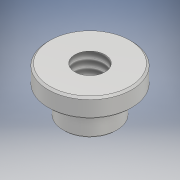
# Autodesk Inventor part: Nut_SMD_M2x0.4_1mm
Saved by Autodesk Inventor 2018 (Build 220112000, 112)
## iProperties
Created: 2018-10-26
Part Number: Nut_SMD_M2x0.4_1mm
Material: Steel, Mild
Description: 9774010243R
Document SubType Name: Modeling
Designer: Bradley
Density: 7.85 g/cm^3
Appearance: Semi-Polished
Author: Bradley
Autodesk Inventor part; units mm, degrees
ref_plane "YZ Plane" through (0, 0, 0) normal (1, 0, 0) x (0, 1, 0)
ref_plane "XZ Plane" through (0, 0, 0) normal (0, 1, 0) x (-1, 0, 0)
ref_plane "XY Plane" through (0, 0, 0) normal (0, 0, 1) x (1, 0, 0)
sketch "Sketch1" plane through (0, 0, 0) normal (0, 1, 0) x (-1, 0, 0)
  line L0 (0, 1.2) -> (0, -1.2)
  line L1 (0, -1.2) -> (-1.4, -1.2)
  line L2 (-1.4, -1.2) -> (-1.4, 0.2)
  line L3 (-1.4, 0.2) -> (-2.175, 0.2)
  line L4 (-2.175, 0.2) -> (-2.175, 1.2)
  line L5 (-2.175, 1.2) -> (0, 1.2)
  point P0 (0, 0)
  point P1 (0, 0)
  dimension "d1" = 1
  dimension "d2" = 1.4
  dimension "d3" = 2.8
  dimension "d4" = 4.35
  constraints: 14 end point, 4 perpendicular, 1 coincident, 1 midpoint, 1 vertical
  measures "d1" distance of L3.end L4.end
  measures "d2" distance of L1.end L2.end
  measures "d3" diameter of L2 L0
  measures "d4" diameter of L4 L0
revolve "Revolution1" add sketch "Sketch1" angle 360 about axis through (0, 0, 1.2) along (0, 0, -1)
hole "Hole1" at (0, 0, 1.2) direction (0, 0, -1) diameter 1.567 end through all thread size "M2x0.4" class "6H" standard "ANSI Metric M Profile"
chamfer "Chamfer1" distance 0.1 angle 45 3 edges at (-2.175, 0, 1.2) (-2.175, 0, 0.2) (-1.4, 0, -1.2)
body "Solid1"
